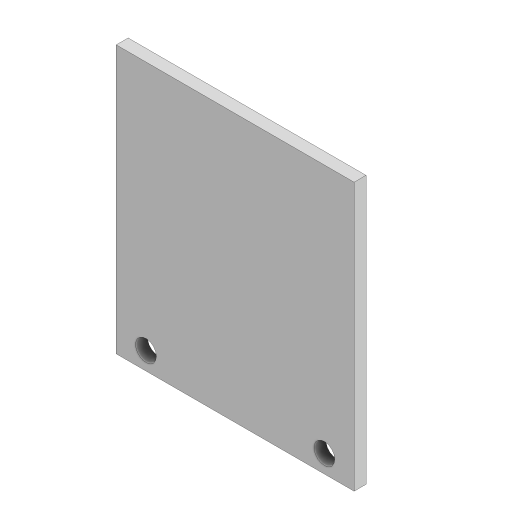
# Autodesk Inventor part: HOLDER_MARKER_ROBOTAT
Saved by Autodesk Inventor 2024.2 (Build 282272000, 272)
## iProperties
Created: 2023-09-22
Part Number: HOLDER_MARKER_ROBOTAT
Material: Generic
Document SubType Name: Modeling
Designer: jalva
Density: 1 g/cm^3
Appearance: Default
Author: jalva
Autodesk Inventor part; units mm, degrees
ref_plane "YZ Plane" through (0, 0, 0) normal (1, 0, 0) x (0, 1, 0)
ref_plane "XZ Plane" through (0, 0, 0) normal (0, 1, 0) x (-1, 0, 0)
ref_plane "XY Plane" through (0, 0, 0) normal (0, 0, 1) x (1, 0, 0)
sketch "Sketch1" plane through (0, 0, 0) normal (0, 0, 1) x (1, 0, 0)
  line L0 (0, 0) -> (40, 0)
  line L1 (40, 0) -> (40, 45)
  line L2 (40, 45) -> (0, 45)
  line L3 (0, 45) -> (0, 0)
  circle A0 centre (5, 3) radius 1.75
  circle A1 centre (12.5, 3) radius 1.75
  circle A2 centre (20, 3) radius 1.75
  circle A3 centre (27.5, 3) radius 1.75
  circle A4 centre (35, 3) radius 1.75
  line L4 (7.5, 17.5) -> (32.5, 17.5)
  line L5 (32.5, 17.5) -> (32.5, 37.5)
  line L6 (32.5, 37.5) -> (7.5, 37.5)
  line L7 (7.5, 37.5) -> (7.5, 17.5)
  line L8 (7.5, 17.5) -> (32.5, 37.5) construction
  line L9 (32.5, 17.5) -> (7.5, 37.5) construction
  circle A5 centre (32.5, 37.5) radius 2
  circle A6 centre (32.5, 17.5) radius 2
  circle A7 centre (7.5, 17.5) radius 2
  circle A8 centre (7.5, 37.5) radius 2
  point P0 (20, 45)
  point P1 (20, 27.5)
  point P2 (40, 22.5)
  dimension "d0" = 3.5
  dimension "d3" = 7.5
  dimension "d8" = 40
  dimension "d9" = 45
  dimension "d10" = 4
  dimension "d11" = 4
  dimension "d12" = 4
  dimension "d13" = 4
  dimension "d14" = 20
  dimension "d15" = 25
  dimension "d16" = 5
  dimension "d21" = 3
  constraints: 20 end point, 9 centre point, 4 coincident, 4 midpoint, 4 parallel, 3 horizontal, 2 perpendicular, 2 vertical alignment, 8 other
  measures "d0" diameter of A0
  measures "d3" distance of A0.centre A1.centre
  measures "d8" distance of L1.end L2.end
  measures "d9" distance of L0.end L1.end
  measures "d10" diameter of A5
  measures "d11" diameter of A6
  measures "d12" diameter of A7
  measures "d13" diameter of A8
  measures "d14" distance of L4.end L5.end
  measures "d15" distance of L5.end L6.end
  measures "d16" vertical distance of point (20, 27.5) point (40, 22.5)
  measures "d21" distance from line of L0 A4.centre
extrude "Extrusion1" add sketch "Sketch1" along normal blind 2 contours L3 L2 L1 L0 | A1 | A2 | A3 | L7 A7 L4 | L4 A7 L7 | A7 L7 A8 L6 A5 L5 A6 L4 | A6 L5 L4 | L4 L5 A6 | A8 L6 L7 | L7 L6 A8 | A5 L6 L5 | L5 L6 A5
extrude "Extrusion2" add sketch "Sketch1" against normal blind 5 contours L7 A7 L4 | L4 A7 L7 | A6 L5 L4 | L4 L5 A6 | A8 L6 L7 | L7 L6 A8 | A5 L6 L5 | L5 L6 A5
body "Solid1"
